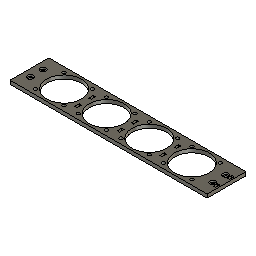
rear_fan_plate (Autodesk Fusion 360 design; units mm, degrees)
part number: 2026-08-23-15-29-27-586
Autodesk Fusion 360 part; units mm, degrees
sketch "Sketch1" plane through (0, 0, 0) normal (0, 0, 1) x (1, 0, 0)
  line L0 (-111, 0.4) -> (111, 0.4)
  line L1 (111, 0.4) -> (111, 44.05)
  line L2 (111, 44.05) -> (-111, 44.05)
  line L3 (-111, 44.05) -> (-111, 0.4)
extrude "Extrude1" add sketch "Sketch1" along normal blind 4
sketch "Sketch2" plane through (0, 0, 0) normal (0, 0, 1) x (1, 0, 0)
  circle A0 centre (-72, 22.225) radius 19.5
  circle A1 centre (-88, 6.225) radius 1.8
  circle A2 centre (-88, 38.225) radius 1.8
  circle A3 centre (-56, 6.225) radius 1.8
  circle A4 centre (-56, 38.225) radius 1.8
  circle A5 centre (-24, 22.225) radius 19.5
  circle A6 centre (-40, 6.225) radius 1.8
  circle A7 centre (-40, 38.225) radius 1.8
  circle A8 centre (-8, 6.225) radius 1.8
  circle A9 centre (-8, 38.225) radius 1.8
  circle A10 centre (24, 22.225) radius 19.5
  circle A11 centre (8, 6.225) radius 1.8
  circle A12 centre (8, 38.225) radius 1.8
  circle A13 centre (40, 6.225) radius 1.8
  circle A14 centre (40, 38.225) radius 1.8
  circle A15 centre (72, 22.225) radius 19.5
  circle A16 centre (56, 6.225) radius 1.8
  circle A17 centre (56, 38.225) radius 1.8
  circle A18 centre (88, 6.225) radius 1.8
  circle A19 centre (88, 38.225) radius 1.8
  circle A20 centre (-102.82, 15) radius 1.7
  circle A21 centre (-102.82, 29.45) radius 1.7
  circle A22 centre (102.82, 15) radius 1.7
  circle A23 centre (102.82, 29.45) radius 1.7
extrude "Extrude2" cut sketch "Sketch2" along normal blind 4
sketch "Sketch3" plane through (0, 0, 0) normal (0, 0, 1) x (1, 0, 0)
  line L0 (-49.25, 11.5) -> (-46.75, 11.5)
  line L1 (-46.75, 11.5) -> (-46.75, 16.5)
  line L2 (-46.75, 16.5) -> (-49.25, 16.5)
  line L3 (-49.25, 16.5) -> (-49.25, 11.5)
  line L4 (-49.25, 27.5) -> (-46.75, 27.5)
  line L5 (-46.75, 27.5) -> (-46.75, 32.5)
  line L6 (-46.75, 32.5) -> (-49.25, 32.5)
  line L7 (-49.25, 32.5) -> (-49.25, 27.5)
  line L8 (-1.25, 11.5) -> (1.25, 11.5)
  line L9 (1.25, 11.5) -> (1.25, 16.5)
  line L10 (1.25, 16.5) -> (-1.25, 16.5)
  line L11 (-1.25, 16.5) -> (-1.25, 11.5)
  line L12 (-1.25, 27.5) -> (1.25, 27.5)
  line L13 (1.25, 27.5) -> (1.25, 32.5)
  line L14 (1.25, 32.5) -> (-1.25, 32.5)
  line L15 (-1.25, 32.5) -> (-1.25, 27.5)
  line L16 (46.75, 11.5) -> (49.25, 11.5)
  line L17 (49.25, 11.5) -> (49.25, 16.5)
  line L18 (49.25, 16.5) -> (46.75, 16.5)
  line L19 (46.75, 16.5) -> (46.75, 11.5)
  line L20 (46.75, 27.5) -> (49.25, 27.5)
  line L21 (49.25, 27.5) -> (49.25, 32.5)
  line L22 (49.25, 32.5) -> (46.75, 32.5)
  line L23 (46.75, 32.5) -> (46.75, 27.5)
  line L24 (106.75, 11.5) -> (109.25, 11.5)
  line L25 (109.25, 11.5) -> (109.25, 16.5)
  line L26 (109.25, 16.5) -> (106.75, 16.5)
  line L27 (106.75, 16.5) -> (106.75, 11.5)
  line L28 (106.75, 27.5) -> (109.25, 27.5)
  line L29 (109.25, 27.5) -> (109.25, 32.5)
  line L30 (109.25, 32.5) -> (106.75, 32.5)
  line L31 (106.75, 32.5) -> (106.75, 27.5)
extrude "Extrude3" cut sketch "Sketch3" along normal blind 4
ref_plane "WorkPlane1" through (0, 0, 4) normal (0, 0, 1) x (1, 0, 0)
sketch "Sketch4" plane through (0, 0, 4) normal (0, 0, 1) x (1, 0, 0)
  circle A0 centre (-102.82, 15) radius 3.25
  circle A1 centre (-102.82, 29.45) radius 3.25
  circle A2 centre (102.82, 15) radius 3.25
  circle A3 centre (102.82, 29.45) radius 3.25
extrude "Extrude4" cut sketch "Sketch4" against normal blind 2
named bodies: "Rear Fan Plate"
